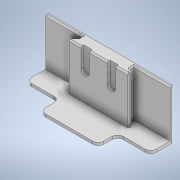
# Autodesk Inventor part: EndSwitchMountingPlate_v02
Saved by Autodesk Inventor 2020 (Build 240168000, 168)
## iProperties
Created: 2020-02-12
Part Number: EndSwitchMountingPlate_v02
Material: Generic
Document SubType Name: Modeling
Designer: Timo
Density: 1 g/cm^3
Appearance: Default
Author: Timo
Autodesk Inventor part; units mm, degrees
ref_plane "YZ Plane" through (0, 0, 0) normal (1, 0, 0) x (0, 1, 0)
ref_plane "XZ Plane" through (0, 0, 0) normal (0, 1, 0) x (-1, 0, 0)
ref_plane "XY Plane" through (0, 0, 0) normal (0, 0, 1) x (1, 0, 0)
sketch "Sketch1" plane through (0, 0, 0) normal (0, 0, 1) x (1, 0, 0)
  line L0 (-22.5, 18) -> (22.5, 18)
  line L1 (22.5, 18) -> (22.5, 0)
  line L2 (22.5, 0) -> (-22.5, 0)
  line L3 (-22.5, 0) -> (-22.5, 18)
  point P0 (0, 0)
  point P1 (0, 0)
  dimension "d0" = 18
  dimension "d1" = 45
  constraints: 8 end point, 2 parallel, 1 coincident, 1 horizontal, 1 midpoint, 1 perpendicular
  measures "d0" distance of L0.end L1.end
  measures "d1" distance of L0.start L0.end
extrude "Extrusion1" add sketch "Sketch1" along normal blind 1
sketch "Sketch2" plane through (0, 0, 1) normal (0, 0, 1) x (1, 0, 0)
  line L0 (-22.5, 18) -> (-22.5, 0) projected
  line L1 (-22.5, 0) -> (22.5, 0) projected
  line L2 (-10.5, 1) -> (10.5, 1)
  line L3 (10.5, 1) -> (10.5, 0)
  line L4 (10.5, 0) -> (-10.5, 0)
  line L5 (-10.5, 0) -> (-10.5, 1)
  point P0 (0, 0)
  point P1 (0, 0)
  dimension "d28" = 21
  dimension "d29" = 1
  constraints: 8 end point, 2 midpoint, 2 parallel, 1 horizontal, 1 perpendicular, 1 point on line
  measures "d28" distance of L2.start L2.end
  measures "d29" distance of L2.end L3.end
extrude "Extrusion2" add sketch "Sketch2" along normal blind 14
sketch "Sketch5" plane through (0, 0, 1) normal (0, 0, 1) x (1, 0, 0)
  line L0 (-22.5, 0) -> (22.5, 0) projected
  line L1 (-22.5, 18) -> (-22.5, 0) projected
  line L2 (22.5, 0) -> (-22.5, 0)
  line L3 (-22.5, 0) -> (-22.5, 1)
  line L4 (-22.5, 1) -> (22.5, 1)
  line L5 (22.5, 1) -> (22.5, 0)
  line L6 (10.5, 1) -> (-10.5, 1) projected
  constraints: 8 end point, 2 parallel, 1 collinear, 1 horizontal, 1 perpendicular, 1 point on line
extrude "Extrusion5" add sketch "Sketch5" along normal blind 7
sketch "Sketch3" plane through (-22.5, 18, 0) normal (0, 1, 0) x (1, 0, 0)
  line L0 (45, -1) -> (0, -1) projected
  line L1 (13.1, -1) -> (13.1, -2.1)
  line L2 (13.1, -2.1) -> (11.6, -3.6)
  line L3 (11.6, -3.6) -> (11.6, -4.5)
  line L4 (11.6, -4.5) -> (33.4, -4.5)
  line L5 (33.4, -4.5) -> (33.4, -3.6)
  line L6 (33.4, -3.6) -> (31.9, -2.1)
  line L7 (31.9, -2.1) -> (31.9, -1)
  line L8 (7, -1) -> (43, -1) projected
  line L9 (22.5, 3) -> (22.5, -18) projected
  point P0 (22.5, 0)
  dimension "d11" = 135
  dimension "d12" = 1.1
  dimension "d13" = 0.9
  dimension "d14" = 21.8
  dimension "d15" = 3.5
  dimension "d27" = 18.8
  constraints: 14 end point, 3 parallel, 3 perpendicular, 2 point on line, 1 vertical, 2 other
  measures "d11" angle of L2 L1
  measures "d12" distance of L1.start L1.end
  measures "d13" distance of L2.end L3.end
  measures "d14" distance of L3.end L4.end
  measures "d15" distance between parallel lines of L0 L4
  measures "d27" distance between parallel lines of L7 L1
extrude "Extrusion3" add sketch "Sketch3" against normal up to surface (18 mm away)
chamfer "Chamfer1" distance 0.5 angle 45 9 edges at (0, 18, 4.5) (10.9, 18, 4.05) (10.15, 18, 2.85) (9.4, 18, 1.55) (15.95, 18, 1) (-10.9, 18, 4.05) (-10.15, 18, 2.85) (-9.4, 18, 1.55) (-15.95, 18, 1)
fillet "Fillet1" radius 0.4 2 edges at (10.9, 9.25, 4.5) (-10.9, 9.25, 4.5)
fillet "Fillet1" radius 0.5 2 edges at (22.5, 9, 0) (-22.5, 9, 0)
sketch "Sketch6" plane through (-10.4, 18, 4) normal (0, 1, 0) x (1, 0, 0)
  line L0 (4.15, -8.7835) -> (7.15, -8.7835)
  line L1 (7.15, -8.7835) -> (7.15, 0.5)
  line L2 (7.15, 0.5) -> (4.15, 0.5)
  line L3 (4.15, 0.5) -> (4.15, -8.7835)
  line L4 (13.65, -8.7835) -> (16.65, -8.7835)
  line L5 (16.65, -8.7835) -> (16.65, 0.5)
  line L6 (16.65, 0.5) -> (13.65, 0.5)
  line L7 (13.65, 0.5) -> (13.65, -8.7835)
  line L8 (5.65, -8.7835) -> (5.65, 0.5) construction
  line L9 (15.15, 0.5) -> (15.15, -8.7835) construction
  line L10 (-0.1, -0.5) -> (20.9, -0.5) construction
  point P0 (10.4, 4)
  dimension "d30" = 3
  dimension "d31" = 1
  dimension "d32" = 9.5
  dimension "d33" = 4.75
  constraints: 20 end point, 4 midpoint, 4 parallel, 2 horizontal, 2 perpendicular, 2 point on line, 1 collinear
  measures "d30" distance of L1.end L2.end
  measures "d31" distance from line of L8.end L10
  measures "d32" distance between parallel lines of L9 L8
  measures "d33" distance from line of L8 point (10.4, 4)
extrude "Extrusion6" cut sketch "Sketch6" against normal blind 7
sketch "Sketch7" plane through (-10.5, 1, 4.5) normal (0, 0, 1) x (1, 0, 0)
  line L0 (7.25, 10) -> (4.25, 10) projected
  arc A0 (4.25, 10) -> (7.25, 10) centre (5.75, 10) ccw
  line L1 (16.75, 10) -> (13.75, 10) projected
  arc A1 (13.75, 10) -> (16.75, 10) centre (15.25, 10) ccw
  line L2 (7.25, 16.5) -> (7.25, 10) projected
  line L3 (13.75, 10) -> (13.75, 16.5) projected
  point P0 (10.5, -1)
  constraints: 4 point on circle, 2 centre point, 2 tangent
extrude "Extrusion7" cut sketch "Sketch7" against normal up to surface (1 mm away)
fillet "Fillet2" radius 2 6 edges at (10.5, 0.5, 8) (22.5, 0.5, 8) (-22.5, 0.5, 8) (-10.5, 0.5, 8) (-10.5, 0.5, 15) (10.5, 0.5, 15)
equation "\"d33\" = 0.5 * d32"
body "Solid1"
